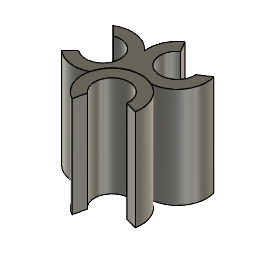
PunchHolderV2 (Autodesk Fusion 360 design; units mm, degrees)
Autodesk Fusion 360 part; units mm, degrees
sketch "Sketch1" plane through (0, 0, 0) normal (0, 0, 1) x (1, 0, 0)
  circle A0 centre (0, 0) radius 4.3
  circle A1 centre (0, 0) radius 7.3
  line L0 (-3.8235, 1.9675) -> (-6.2809, 3.7202)
  line L1 (3.7566, 2.0923) -> (5.4718, 4.8321)
  dimension "d5" = 8.6
  dimension "d9" = 3
  constraint coincident A0.centre A1.centre
  constraint coincident A0 L0.start
  constraint coincident A1 L0.end
  constraint coincident A0 L1.start
  constraint coincident A1 L1.end
  measures "d5" diameter of A0
extrude "Extrude1" add sketch "Sketch1" along normal blind 25 contours A0 A1 L0 L1 picked at (-5.6209, 2.8158) makes body 1
copy_body "CopyPasteBodies1" bodies 1 makes body 2
move_body "Move1" bodies 2 to x (-0.939693, -0.34202, 0) y (0.34202, -0.939693, 0) z (0, 0, 1) at (-2.5077, -12.8055, 0)
copy_body "CopyPasteBodies2" bodies 2 makes body 3
move_body "Move2" bodies 3 to x (-0.5, -0.866025, 0) y (0.866025, -0.5, 0) z (0, 0, 1) at (-3.0916, -13.1494, -0.0571)
move_body "Move3" bodies 1 to x (0.906308, -0.422618, 0) y (0.422618, 0.906308, 0) z (0, 0, 1) at (-0.1394, 1.1103, -0.0571)
sketch "Sketch2" plane through (0, 0, 24.9429) normal (0, 0, 1) x (-1, 0, 0)
  arc A0 (2.7732, -4.5093) -> (-4.1495, -1.419) centre (0.1394, -1.1103) ccw
  line L0 (2.7732, -4.5093) -> (4.2596, -7.1364)
  arc A1 (4.2596, -7.1364) -> (-6.8619, -3.1772) centre (0.1394, -1.1103) ccw
  line L1 (8.0267, 2.5322) -> (3.1056, 2.5322)
  line L2 (3.1056, 2.5322) -> (3.1056, 7.6445)
  line L3 (3.1056, 7.6445) -> (8.0267, 7.6445)
  line L4 (8.0267, 7.6445) -> (8.0267, 2.5322)
  line L5 (-6.8619, -3.1772) -> (-4.1495, -1.419)
  constraint horizontal L1
  constraint vertical L2
  constraint horizontal L3
  constraint vertical L4
extrude "Extrude2" add sketch "Sketch2" against normal blind 25 contours A1 L1 L2 | A1 L1 L2 L3 L4 bodies 1 2 3
equation "PunchDiameter = 8.6 mm"
equation "PunchLength = 25 mm"
equation "d5 = PunchDiameter"
equation "d6 = PunchLength"
equation "GrabberWidth = 3 mm"
equation "d9 = GrabberWidth"
